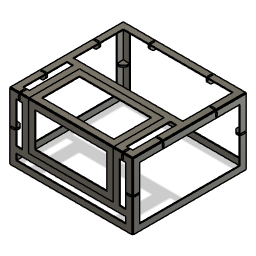
Frameoko_V1.0.0 (Autodesk Fusion 360 design; units mm, degrees)
Autodesk Fusion 360 part; units mm, degrees
(part 1 of 3)
sketch "machine_footprint" plane through (0, 0, 0) normal (0, 1, 0) x (1, 0, 0)
  line L0 (495.3, 457.2) -> (-495.3, 457.2)
  line L1 (-495.3, 457.2) -> (-495.3, -457.2)
  line L2 (-495.3, -457.2) -> (495.3, -457.2)
  line L3 (495.3, -457.2) -> (495.3, 457.2)
  line L4 (495.3, 457.2) -> (-495.3, -457.2) construction
  line L5 (-495.3, 457.2) -> (495.3, -457.2) construction
  dimension "d4" = 990.6
  dimension "d5" = 914.4
  constraint horizontal L0
  constraint perpendicular L0 L1
  constraint parallel L0 L2
  constraint parallel L1 L3
  constraint coincident L4 origin
  constraint coincident L5 origin
  measures "d4" distance of L1.end L2.end
  measures "d5" distance of L0.end L1.end
extrude "Extrude1" add sketch "machine_footprint" along normal mid plane 533.4 makes body 1
sketch "back-face" plane through (0, 0, 0) normal (0, 0, 1) x (1, 0, 0)
  line L0 (495.3, 266.7) -> (-495.3, 266.7)
  line L1 (-495.3, 266.7) -> (-495.3, -266.7)
  line L2 (-495.3, -266.7) -> (495.3, -266.7)
  line L3 (495.3, -266.7) -> (495.3, 266.7)
  line L4 (495.3, 266.7) -> (-495.3, -266.7) construction
  line L5 (-495.3, 266.7) -> (495.3, -266.7) construction
  line L6 (444.5, 215.9) -> (-444.5, 215.9)
  line L7 (-444.5, 215.9) -> (-444.5, -215.9)
  line L8 (-444.5, -215.9) -> (444.5, -215.9)
  line L9 (444.5, -215.9) -> (444.5, 215.9)
  line L10 (444.5, 215.9) -> (-444.5, -215.9) construction
  line L11 (-444.5, 215.9) -> (444.5, -215.9) construction
  line L12 (-495.3, 266.7) -> (-444.5, 266.7)
  line L13 (-444.5, 266.7) -> (-444.5, 215.9)
  line L14 (-444.5, 215.9) -> (-495.3, 215.9)
  line L15 (-495.3, 215.9) -> (-495.3, 266.7)
  line L16 (495.3, 266.7) -> (444.5, 266.7)
  line L17 (444.5, 266.7) -> (444.5, 215.9)
  line L18 (444.5, 215.9) -> (495.3, 215.9)
  line L19 (495.3, 215.9) -> (495.3, 266.7)
  line L20 (495.3, -266.7) -> (444.5, -266.7)
  line L21 (444.5, -266.7) -> (444.5, -215.9)
  line L22 (444.5, -215.9) -> (495.3, -215.9)
  line L23 (495.3, -215.9) -> (495.3, -266.7)
  line L24 (-495.3, -266.7) -> (-444.5, -266.7)
  line L25 (-444.5, -266.7) -> (-444.5, -215.9)
  line L26 (-444.5, -215.9) -> (-495.3, -215.9)
  line L27 (-495.3, -215.9) -> (-495.3, -266.7)
  line L28 (-444.5, 266.7) -> (-444.5, 215.9)
  line L29 (-444.5, 215.9) -> (-393.7, 215.9)
  line L30 (-393.7, 215.9) -> (-393.7, 266.7)
  line L31 (-393.7, 266.7) -> (-444.5, 266.7)
  line L32 (444.5, 266.7) -> (444.5, 215.9)
  line L33 (444.5, 215.9) -> (393.7, 215.9)
  line L34 (393.7, 215.9) -> (393.7, 266.7)
  line L35 (393.7, 266.7) -> (444.5, 266.7)
  line L36 (-444.5, 215.9) -> (-495.3, 215.9)
  line L37 (-495.3, 215.9) -> (-495.3, 165.1)
  line L38 (-495.3, 165.1) -> (-444.5, 165.1)
  line L39 (-444.5, 165.1) -> (-444.5, 215.9)
  line L40 (495.3, 215.9) -> (444.5, 215.9)
  line L41 (444.5, 215.9) -> (444.5, 165.1)
  line L42 (444.5, 165.1) -> (495.3, 165.1)
  line L43 (495.3, 165.1) -> (495.3, 215.9)
  line L44 (495.3, -215.9) -> (444.5, -215.9)
  line L45 (444.5, -215.9) -> (444.5, -165.1)
  line L46 (444.5, -165.1) -> (495.3, -165.1)
  line L47 (495.3, -165.1) -> (495.3, -215.9)
  line L48 (444.5, -215.9) -> (444.5, -266.7)
  line L49 (444.5, -266.7) -> (393.7, -266.7)
  line L50 (393.7, -266.7) -> (393.7, -215.9)
  line L51 (393.7, -215.9) -> (444.5, -215.9)
  line L52 (-444.5, -215.9) -> (-444.5, -266.7)
  line L53 (-444.5, -266.7) -> (-393.7, -266.7)
  line L54 (-393.7, -266.7) -> (-393.7, -215.9)
  line L55 (-393.7, -215.9) -> (-444.5, -215.9)
  line L56 (-444.5, -215.9) -> (-495.3, -215.9)
  line L57 (-495.3, -215.9) -> (-495.3, -165.1)
  line L58 (-495.3, -165.1) -> (-444.5, -165.1)
  line L59 (-444.5, -165.1) -> (-444.5, -215.9)
  line L60 (444.5, 266.7) -> (393.7, 215.9)
  line L61 (495.3, 215.9) -> (444.5, 165.1)
  line L62 (495.3, -215.9) -> (444.5, -165.1)
  line L63 (393.7, -215.9) -> (444.5, -266.7)
  line L64 (-444.5, -266.7) -> (-393.7, -215.9)
  line L65 (-495.3, -215.9) -> (-444.5, -165.1)
  line L66 (-444.5, 266.7) -> (-393.7, 215.9)
  line L67 (-495.3, 215.9) -> (-444.5, 165.1)
  circle A0 centre (-419.1, 241.3) radius 15.875
  circle A1 centre (419.1, 241.3) radius 15.875
  circle A2 centre (469.9, 190.5) radius 15.875
  circle A3 centre (469.9, -190.5) radius 15.875
  circle A4 centre (419.1, -241.3) radius 15.875
  circle A5 centre (-419.1, -241.3) radius 15.875
  circle A6 centre (-469.9, -190.5) radius 15.875
  circle A7 centre (-469.9, 190.5) radius 15.875
  line L68 (-165.1, 266.7) -> (-165.1, 215.9)
  circle A8 centre (-139.7, 241.3) radius 15.875
  line L69 (-114.3, 215.9) -> (-114.3, 266.7)
  line L70 (114.3, 266.7) -> (114.3, 215.9)
  circle A9 centre (139.7, 241.3) radius 15.875
  line L71 (165.1, 215.9) -> (165.1, 266.7)
  circle A10 centre (469.9, -190.5) radius 15.875
  line L72 (495.3, -165.1) -> (444.5, -165.1)
  line L73 (444.5, -215.9) -> (495.3, -215.9)
  line L74 (393.7, 266.7) -> (393.7, 215.9)
  circle A11 centre (419.1, 241.3) radius 15.875
  line L75 (444.5, 215.9) -> (444.5, 266.7)
  circle A12 centre (-469.9, -190.5) radius 15.875
  line L76 (-495.3, -215.9) -> (-444.5, -215.9)
  line L77 (-444.5, -165.1) -> (-495.3, -165.1)
  circle A13 centre (-139.7, -241.3) radius 15.875
  line L78 (-114.3, -266.7) -> (-114.3, -215.9)
  line L79 (-165.1, -266.7) -> (-165.1, -215.9)
  circle A14 centre (139.7, -241.3) radius 15.875
  line L80 (165.1, -266.7) -> (165.1, -215.9)
  line L81 (114.3, -266.7) -> (114.3, -215.9)
  circle A15 centre (419.1, -241.3) radius 15.875
  line L82 (444.5, -266.7) -> (444.5, -215.9)
  line L83 (393.7, -266.7) -> (393.7, -215.9)
  dimension "d49" = 990.6
  dimension "d50" = 533.4
  dimension "d51" = 889
  dimension "d52" = 431.8
  dimension "d259" = 50.8
  dimension "d260" = 50.8
  dimension "d261" = 50.8
  dimension "d262" = 50.8
  dimension "d263" = 50.8
  dimension "d264" = 50.8
  dimension "d265" = 50.8
  dimension "d266" = 50.8
  dimension "d267" = 50.8
  dimension "d268" = 50.8
  dimension "d269" = 50.8
  dimension "d270" = 50.8
  dimension "d271" = 50.8
  dimension "d272" = 50.8
  dimension "d273" = 50.8
  dimension "d274" = 50.8
  dimension "d275" = 31.75
  dimension "d276" = 31.75
  dimension "d277" = 31.75
  dimension "d278" = 31.75
  dimension "d279" = 31.75
  dimension "d280" = 31.75
  dimension "d281" = 31.75
  dimension "d282" = 31.75
  dimension "d285" = 838.2
  dimension "d286" = 0
  dimension "d297" = 0
  dimension "d298" = -381
  constraint horizontal L0
  constraint perpendicular L0 L1
  constraint parallel L0 L2
  constraint parallel L1 L3
  constraint coincident L4 origin
  constraint coincident L5 origin
  constraint horizontal L6
  constraint perpendicular L6 L7
  constraint parallel L6 L8
  constraint parallel L7 L9
  constraint coincident L10 origin
  constraint coincident L11 origin
  constraint horizontal L12
  constraint vertical L13
  constraint horizontal L14
  constraint vertical L15
  constraint horizontal L16
  constraint vertical L17
  constraint horizontal L18
  constraint vertical L19
  constraint horizontal L20
  constraint vertical L21
  constraint horizontal L22
  constraint vertical L23
  constraint horizontal L24
  constraint vertical L25
  constraint horizontal L26
  constraint vertical L27
  constraint perpendicular L28 L29
  constraint parallel L28 L30
  constraint parallel L29 L31
  constraint perpendicular L32 L33
  constraint parallel L32 L34
  constraint parallel L33 L35
  constraint perpendicular L36 L37
  constraint parallel L36 L38
  constraint parallel L37 L39
  constraint perpendicular L40 L41
  constraint parallel L40 L42
  constraint parallel L41 L43
  constraint perpendicular L44 L45
  constraint parallel L44 L46
  constraint parallel L45 L47
  constraint perpendicular L48 L49
  constraint parallel L48 L50
  constraint parallel L49 L51
  constraint perpendicular L52 L53
  constraint parallel L52 L54
  constraint parallel L53 L55
  constraint perpendicular L56 L57
  constraint parallel L56 L58
  constraint parallel L57 L59
  constraint midpoint L66 A0.centre
  constraint midpoint L60 A1.centre
  constraint midpoint L61 A2.centre
  constraint midpoint L62 A3.centre
  constraint midpoint L63 A4.centre
  constraint midpoint L64 A5.centre
  constraint midpoint L65 A6.centre
  constraint midpoint L67 A7.centre
  measures "d49" distance of L1.end L2.end
  measures "d50" distance of L0.end L1.end
  measures "d51" distance of L7.end L8.end
  measures "d52" distance of L6.end L7.end
  measures "d259" distance of L0.end L12.end
  measures "d260" distance of L0.end L14.end
  measures "d261" distance of L0.start L16.end
  measures "d262" distance of L0.start L18.end
  measures "d263" distance of L2.end L20.end
  measures "d264" distance of L2.end L22.end
  measures "d265" distance of L1.end L24.end
  measures "d266" distance of L1.end L26.end
  measures "d267" distance of L12.end L30.end
  measures "d268" distance of L16.end L34.end
  measures "d269" distance of L6.end L38.end
  measures "d270" distance of L18.end L42.end
  measures "d271" distance of L22.end L46.end
  measures "d272" distance of L8.end L50.end
  measures "d273" distance of L7.end L54.end
  measures "d274" distance of L7.end L58.end
  measures "d275" diameter of A0
  measures "d276" diameter of A1
  measures "d277" diameter of A2
  measures "d278" diameter of A3
  measures "d279" diameter of A4
  measures "d280" diameter of A5
  measures "d281" diameter of A6
  measures "d282" diameter of A7
extrude "Extrude9" add sketch "back-face" along normal blind -457.2 and the other way blind 463.55 separate body contours L0 L3 L16 L17 L18 L19 L32 L40 L75 | L0 L34 L35 L60 A1 L74 A11 | L6 L17 L32 L33 L60 A1 A11 L75 | L9 L18 L40 L41 L61 A2 | L3 L42 L43 L61 A2 | L0 L6 L34 L71 L74 | L60 A1 A11 | L60 A1 A11 | L3 L9 L42 L46 L72 | L61 A2 | L61 A2 | L0 L6 L70 L71 | L3 L46 L47 L62 A3 A10 L72 | L0 L6 L69 L70 | L9 L22 L44 L45 L62 A3 A10 L73 | L2 L3 L20 L21 L22 L23 L44 L48 L73 L82 | L0 L6 L68 L69 | L8 L21 L48 L51 L63 A4 A15 L82 | L62 A3 A10 | L62 A3 A10 | L0 L6 L30 L68 | L2 L8 L50 L80 L83 | L2 L49 L50 L63 A4 A15 L83 | L0 L30 L31 L66 A0 | L2 L8 L80 L81 | L63 A4 A15 | L63 A4 A15 | L0 L1 L12 L13 L14 L15 L28 L36 | L6 L13 L28 L29 L66 A0 | L2 L8 L78 L81 | L7 L14 L36 L39 L67 A7 | L66 A0 | L66 A0 | L2 L8 L78 L79 | L1 L37 L38 L67 A7 | L1 L7 L38 L58 L77 | L2 L8 L54 L79 | L67 A7 | L67 A7 | L1 L57 L58 L65 A6 A12 L77 | L7 L26 L56 L59 L65 A6 A12 L76 | L8 L25 L52 L55 L64 A5 | L2 L53 L54 L64 A5 | L1 L2 L24 L25 L26 L27 L52 L56 L76 | L65 A6 A12 | L65 A6 A12 | L64 A5 | L64 A5 | A8 | A9 | A13 | A14 makes body 2
sketch "LR-faces" plane through (0, 0, 0) normal (1, 0, 0) x (0, 0, -1)
  line L0 (457.2, 266.7) -> (-457.2, 266.7)
  line L1 (-457.2, 266.7) -> (-457.2, -266.7)
  line L2 (-457.2, -266.7) -> (457.2, -266.7)
  line L3 (457.2, -266.7) -> (457.2, 266.7)
  line L4 (457.2, 266.7) -> (-457.2, -266.7) construction
  line L5 (-457.2, 266.7) -> (457.2, -266.7) construction
  line L6 (406.4, 215.9) -> (-406.4, 215.9)
  line L7 (-406.4, 215.9) -> (-406.4, -215.9)
  line L8 (-406.4, -215.9) -> (406.4, -215.9)
  line L9 (406.4, -215.9) -> (406.4, 215.9)
  line L10 (406.4, 215.9) -> (-406.4, -215.9) construction
  line L11 (-406.4, 215.9) -> (406.4, -215.9) construction
  line L12 (-457.2, 266.7) -> (-406.4, 266.7)
  line L13 (-406.4, 266.7) -> (-406.4, 215.9)
  line L14 (-406.4, 215.9) -> (-457.2, 215.9)
  line L15 (-457.2, 215.9) -> (-457.2, 266.7)
  line L16 (457.2, 266.7) -> (406.4, 266.7)
  line L17 (406.4, 266.7) -> (406.4, 215.9)
  line L18 (406.4, 215.9) -> (457.2, 215.9)
  line L19 (457.2, 215.9) -> (457.2, 266.7)
  line L20 (457.2, -266.7) -> (406.4, -266.7)
  line L21 (406.4, -266.7) -> (406.4, -215.9)
  line L22 (406.4, -215.9) -> (457.2, -215.9)
  line L23 (457.2, -215.9) -> (457.2, -266.7)
  line L24 (-457.2, -266.7) -> (-406.4, -266.7)
  line L25 (-406.4, -266.7) -> (-406.4, -215.9)
  line L26 (-406.4, -215.9) -> (-457.2, -215.9)
  line L27 (-457.2, -215.9) -> (-457.2, -266.7)
  line L28 (-406.4, 266.7) -> (-406.4, 215.9)
  line L29 (-406.4, 215.9) -> (-355.6, 215.9)
  line L30 (-355.6, 215.9) -> (-355.6, 266.7)
  line L31 (-355.6, 266.7) -> (-406.4, 266.7)
  line L32 (406.4, 266.7) -> (406.4, 215.9)
  line L33 (406.4, 215.9) -> (355.6, 215.9)
  line L34 (355.6, 215.9) -> (355.6, 266.7)
  line L35 (355.6, 266.7) -> (406.4, 266.7)
  line L36 (-406.4, 266.7) -> (-355.6, 215.9)
  circle A0 centre (-381, 241.3) radius 15.875
  line L37 (355.6, 266.7) -> (406.4, 215.9)
  circle A1 centre (381, 241.3) radius 15.875
  circle A2 centre (-127, 241.3) radius 15.875
  line L38 (-101.6, 215.9) -> (-101.6, 266.7)
  line L39 (-152.4, 266.7) -> (-152.4, 215.9)
  line L40 (-406.4, -215.9) -> (-406.4, -266.7)
  line L41 (-406.4, -266.7) -> (-355.6, -266.7)
  line L42 (-355.6, -266.7) -> (-355.6, -215.9)
  line L43 (-355.6, -215.9) -> (-406.4, -215.9)
  line L44 (406.4, -215.9) -> (406.4, -266.7)
  line L45 (406.4, -266.7) -> (355.6, -266.7)
  line L46 (355.6, -266.7) -> (355.6, -215.9)
  line L47 (355.6, -215.9) -> (406.4, -215.9)
  line L48 (355.6, -215.9) -> (406.4, -266.7)
  line L49 (-406.4, -215.9) -> (-355.6, -266.7)
  line L50 (-406.4, 215.9) -> (-457.2, 215.9)
  line L51 (-457.2, 215.9) -> (-457.2, 165.1)
  line L52 (-457.2, 165.1) -> (-406.4, 165.1)
  line L53 (-406.4, 165.1) -> (-406.4, 215.9)
  line L54 (-406.4, -215.9) -> (-457.2, -215.9)
  line L55 (-457.2, -215.9) -> (-457.2, -165.1)
  line L56 (-457.2, -165.1) -> (-406.4, -165.1)
  line L57 (-406.4, -165.1) -> (-406.4, -215.9)
  line L58 (-457.2, 215.9) -> (-406.4, 165.1)
  circle A3 centre (-431.8, 190.5) radius 15.875
  circle A4 centre (-381, -241.3) radius 15.875
  circle A5 centre (381, -241.3) radius 15.875
  line L59 (406.4, 215.9) -> (457.2, 215.9)
  line L60 (457.2, 215.9) -> (457.2, 165.1)
  line L61 (457.2, 165.1) -> (406.4, 165.1)
  line L62 (406.4, 165.1) -> (406.4, 215.9)
  line L63 (457.2, -215.9) -> (406.4, -215.9)
  line L64 (406.4, -215.9) -> (406.4, -165.1)
  line L65 (406.4, -165.1) -> (457.2, -165.1)
  line L66 (457.2, -165.1) -> (457.2, -215.9)
  line L67 (406.4, -165.1) -> (457.2, -215.9)
  circle A6 centre (431.8, -190.5) radius 15.875
  line L68 (406.4, 165.1) -> (457.2, 215.9)
  circle A7 centre (431.8, 190.5) radius 15.875
  line L69 (-406.4, -165.1) -> (-457.2, -215.9)
  circle A8 centre (-431.8, -190.5) radius 15.875
  line L70 (-457.2, -215.9) -> (-406.4, -215.9)
  line L71 (-406.4, -165.1) -> (-457.2, -165.1)
  circle A9 centre (-431.8, -190.5) radius 15.875
  circle A10 centre (-127, -241.3) radius 15.875
  line L72 (-152.4, -215.9) -> (-152.4, -266.7)
  line L73 (-101.6, -266.7) -> (-101.6, -215.9)
  circle A11 centre (431.8, -190.5) radius 15.875
  line L74 (406.4, -165.1) -> (457.2, -165.1)
  line L75 (457.2, -215.9) -> (406.4, -215.9)
  circle A12 centre (127, 241.3) radius 15.875
  line L76 (152.4, 215.9) -> (152.4, 266.7)
  line L77 (101.6, 266.7) -> (101.6, 215.9)
  circle A13 centre (127, -241.3) radius 15.875
  line L78 (101.6, -215.9) -> (101.6, -266.7)
  line L79 (152.4, -266.7) -> (152.4, -215.9)
  circle A14 centre (381, 241.3) radius 15.875
  line L80 (406.4, 215.9) -> (406.4, 266.7)
  line L81 (355.6, 266.7) -> (355.6, 215.9)
  circle A15 centre (381, -241.3) radius 15.875
  line L82 (355.6, -215.9) -> (355.6, -266.7)
  line L83 (406.4, -266.7) -> (406.4, -215.9)
  point P0 (0, 292.1)
  point P1 (431.8, 0)
  point P2 (-431.8, 0)
  dimension "d81" = 914.4
  dimension "d82" = 533.4
  dimension "d83" = 812.8
  dimension "d84" = 431.8
  dimension "d202" = 50.8
  dimension "d203" = 50.8
  dimension "d204" = 50.8
  dimension "d205" = 50.8
  dimension "d206" = 50.8
  dimension "d207" = 50.8
  dimension "d208" = 50.8
  dimension "d209" = 50.8
  dimension "d210" = 50.8
  dimension "d211" = 50.8
  dimension "d212" = 31.75
  dimension "d213" = 31.75
  dimension "d216" = 762
  dimension "d217" = 0
  dimension "d218" = 50.8
  dimension "d219" = 50.8
  dimension "d220" = 50.8
  dimension "d221" = 50.8
  dimension "d222" = 31.75
  dimension "d224" = 31.75
  dimension "d225" = 31.75
  dimension "d226" = 50.8
  dimension "d227" = 50.8
  dimension "d229" = 31.75
  dimension "d230" = 31.75
  dimension "d231" = 31.75
  dimension "d239" = 0
  dimension "d240" = -381
  constraint horizontal L0
  constraint perpendicular L0 L1
  constraint parallel L0 L2
  constraint parallel L1 L3
  constraint coincident L4 origin
  constraint coincident L5 origin
  constraint horizontal L6
  constraint perpendicular L6 L7
  constraint parallel L6 L8
  constraint parallel L7 L9
  constraint coincident L10 origin
  constraint coincident L11 origin
  constraint horizontal L12
  constraint vertical L13
  constraint horizontal L14
  constraint vertical L15
  constraint horizontal L16
  constraint vertical L17
  constraint horizontal L18
  constraint vertical L19
  constraint horizontal L20
  constraint vertical L21
  constraint horizontal L22
  constraint vertical L23
  constraint horizontal L24
  constraint vertical L25
  constraint horizontal L26
  constraint vertical L27
  constraint perpendicular L28 L29
  constraint parallel L28 L30
  constraint parallel L29 L31
  constraint perpendicular L32 L33
  constraint parallel L32 L34
  constraint parallel L33 L35
  constraint midpoint L36 A0.centre
  constraint midpoint L37 A1.centre
  constraint perpendicular L40 L41
  constraint parallel L40 L42
  constraint parallel L41 L43
  constraint perpendicular L44 L45
  constraint parallel L44 L46
  constraint parallel L45 L47
  constraint perpendicular L50 L51
  constraint parallel L50 L52
  constraint parallel L51 L53
  constraint perpendicular L54 L55
  constraint parallel L54 L56
  constraint parallel L55 L57
  constraint midpoint L58 A3.centre
  constraint midpoint L49 A4.centre
  constraint midpoint L48 A5.centre
  constraint perpendicular L59 L60
  constraint parallel L59 L61
  constraint parallel L60 L62
  constraint perpendicular L63 L64
  constraint parallel L63 L65
  constraint parallel L64 L66
  constraint midpoint L67 A6.centre
  constraint midpoint L68 A7.centre
  constraint midpoint L69 A8.centre
  measures "d81" distance of L1.end L2.end
  measures "d82" distance of L0.end L1.end
  measures "d83" distance of L7.end L8.end
  measures "d84" distance of L6.end L7.end
  measures "d202" distance of L0.end L12.end
  measures "d203" distance of L0.end L14.end
  measures "d204" distance of L0.start L16.end
  measures "d205" distance of L0.start L18.end
  measures "d206" distance of L2.end L20.end
  measures "d207" distance of L2.end L22.end
  measures "d208" distance of L1.end L24.end
  measures "d209" distance of L1.end L26.end
  measures "d210" distance of L12.end L30.end
  measures "d211" distance of L16.end L34.end
  measures "d212" diameter of A0
  measures "d213" diameter of A1
  measures "d218" distance of L7.end L42.end
  measures "d219" distance of L8.end L46.end
  measures "d220" distance of L6.end L52.end
  measures "d221" distance of L7.end L56.end
  measures "d222" diameter of A3
  measures "d224" diameter of A4
  measures "d225" diameter of A5
  measures "d226" distance of L6.start L61.end
  measures "d227" distance of L22.end L65.end
  measures "d229" diameter of A6
  measures "d230" diameter of A7
  measures "d231" diameter of A8
extrude "Extrude13" add sketch "LR-faces" along normal blind 501.65 and the other way blind -495.3 separate body contours L0 L3 L16 L17 L18 L19 L32 L59 L80 | L0 L17 L32 L35 L37 A1 A14 L80 | L9 L18 L59 L62 L68 A7 | L3 L60 L61 L68 A7 | L0 L6 L34 L76 L81 | L6 L33 L34 L37 A1 A14 L81 | L3 L9 L61 L65 L74 | L68 A7 | L68 A7 | L0 L6 L76 L77 | L37 A1 A14 | L37 A1 A14 | L3 L65 L66 L67 A6 A11 L74 | L0 L6 L38 L77 | L9 L22 L63 L64 L67 A6 A11 L75 | L2 L3 L20 L21 L22 L23 L44 L63 L75 L83 | L0 L6 L38 L39 | L8 L21 L44 L47 L48 A5 A15 L83 | L67 A6 A11 | L67 A6 A11 | L0 L6 L30 L39 | L2 L8 L46 L79 L82 | L2 L45 L46 L48 A5 A15 L82 | L0 L30 L31 L36 A0 | L2 L8 L78 L79 | L48 A5 A15 | L48 A5 A15 | L0 L1 L12 L13 L14 L15 L28 L50 | L6 L13 L28 L29 L36 A0 | L2 L8 L73 L78 | L7 L14 L50 L53 L58 A3 | L36 A0 | L36 A0 | L2 L8 L72 L73 | L1 L51 L52 L58 A3 | L1 L7 L52 L56 L71 | L2 L8 L42 L72 | L58 A3 | L58 A3 | L1 L55 L56 L69 A8 L71 A9 | L7 L26 L54 L57 L69 A8 L70 A9 | L8 L42 L43 L49 A4 | L2 L25 L40 L41 L49 A4 | L1 L2 L24 L25 L26 L27 L40 L54 L70 | L69 A8 A9 | L69 A8 A9 | L49 A4 | L49 A4 | A2 | A10 | A12 | A13 makes body 3
extrude "Extrude14" add sketch "LR-faces" along normal blind -501.65 and the other way blind 495.3 separate body contours L0 L3 L16 L17 L18 L19 L32 L59 L80 | L0 L17 L32 L35 L37 A1 A14 L80 | L9 L18 L59 L62 L68 A7 | L3 L60 L61 L68 A7 | L0 L6 L34 L76 L81 | L6 L33 L34 L37 A1 A14 L81 | L3 L9 L61 L65 L74 | L68 A7 | L68 A7 | L0 L6 L76 L77 | L37 A1 A14 | L37 A1 A14 | L3 L65 L66 L67 A6 A11 L74 | L0 L6 L38 L77 | L9 L22 L63 L64 L67 A6 A11 L75 | L2 L3 L20 L21 L22 L23 L44 L63 L75 L83 | L0 L6 L38 L39 | L8 L21 L44 L47 L48 A5 A15 L83 | L67 A6 A11 | L67 A6 A11 | L0 L6 L30 L39 | L2 L8 L46 L79 L82 | L2 L45 L46 L48 A5 A15 L82 | L0 L30 L31 L36 A0 | L2 L8 L78 L79 | L48 A5 A15 | L48 A5 A15 | L0 L1 L12 L13 L14 L15 L28 L50 | L6 L13 L28 L29 L36 A0 | L2 L8 L73 L78 | L7 L14 L50 L53 L58 A3 | L36 A0 | L36 A0 | L2 L8 L72 L73 | L1 L51 L52 L58 A3 | L1 L7 L52 L56 L71 | L2 L8 L42 L72 | L58 A3 | L58 A3 | L1 L55 L56 L69 A8 L71 A9 | L7 L26 L54 L57 L69 A8 L70 A9 | L8 L42 L43 L49 A4 | L2 L25 L40 L41 L49 A4 | L1 L2 L24 L25 L26 L27 L40 L54 L70 | L69 A8 A9 | L69 A8 A9 | L49 A4 | L49 A4 | A2 | A10 | A12 | A13 makes body 4
sketch "top-face" plane through (0, 0, 0) normal (0, 1, 0) x (1, 0, 0)
  line L0 (495.3, -457.2) -> (-495.3, -457.2)
  line L1 (-495.3, -457.2) -> (-495.3, 457.2)
  line L2 (-495.3, 457.2) -> (495.3, 457.2)
  line L3 (495.3, 457.2) -> (495.3, -457.2)
  line L4 (495.3, -457.2) -> (-495.3, 457.2) construction
  line L5 (-495.3, -457.2) -> (495.3, 457.2) construction
  line L6 (495.3, -457.2) -> (342.9, -457.2)
  line L7 (342.9, -457.2) -> (342.9, -50.8)
  line L8 (342.9, -50.8) -> (495.3, -50.8)
  line L9 (495.3, -50.8) -> (495.3, -457.2)
  line L10 (-495.3, -457.2) -> (-342.9, -457.2)
  line L11 (-342.9, -457.2) -> (-342.9, -50.8)
  line L12 (-342.9, -50.8) -> (-495.3, -50.8)
  line L13 (-495.3, -50.8) -> (-495.3, -457.2)
  line L14 (-495.3, -50.8) -> (495.3, -50.8)
  line L15 (495.3, -50.8) -> (495.3, 0)
  line L16 (495.3, 0) -> (-495.3, 0)
  line L17 (-495.3, 0) -> (-495.3, -50.8)
  line L18 (-495.3, 457.2) -> (495.3, 457.2)
  line L19 (495.3, 457.2) -> (495.3, 406.4)
  line L20 (495.3, 406.4) -> (-495.3, 406.4)
  line L21 (-495.3, 406.4) -> (-495.3, 457.2)
  line L22 (495.3, -457.2) -> (342.9, -457.2)
  line L23 (342.9, -457.2) -> (342.9, -406.4)
  line L24 (342.9, -406.4) -> (495.3, -406.4)
  line L25 (495.3, -406.4) -> (495.3, -457.2)
  line L26 (-495.3, -457.2) -> (-342.9, -457.2)
  line L27 (-342.9, -457.2) -> (-342.9, -406.4)
  line L28 (-342.9, -406.4) -> (-495.3, -406.4)
  line L29 (-495.3, -406.4) -> (-495.3, -457.2)
  line L30 (495.3, -457.2) -> (495.3, 457.2)
  line L31 (495.3, 457.2) -> (444.5, 457.2)
  line L32 (444.5, 457.2) -> (444.5, -457.2)
  line L33 (444.5, -457.2) -> (495.3, -457.2)
  line L34 (-495.3, 457.2) -> (-495.3, -457.2)
  line L35 (-495.3, -457.2) -> (-444.5, -457.2)
  line L36 (-444.5, -457.2) -> (-444.5, 457.2)
  line L37 (-444.5, 457.2) -> (-495.3, 457.2)
  line L38 (-342.9, -457.2) -> (-342.9, -50.8)
  line L39 (-342.9, -50.8) -> (-393.7, -50.8)
  line L40 (-393.7, -50.8) -> (-393.7, -457.2)
  line L41 (-393.7, -457.2) -> (-342.9, -457.2)
  line L42 (342.9, -457.2) -> (342.9, -50.8)
  line L43 (342.9, -50.8) -> (393.7, -50.8)
  line L44 (393.7, -50.8) -> (393.7, -457.2)
  line L45 (393.7, -457.2) -> (342.9, -457.2)
  line L46 (-342.9, -457.2) -> (342.9, -457.2)
  line L47 (342.9, -457.2) -> (342.9, -406.4)
  line L48 (342.9, -406.4) -> (-342.9, -406.4)
  line L49 (-342.9, -406.4) -> (-342.9, -457.2)
  line L50 (-342.9, -50.8) -> (342.9, -50.8)
  line L51 (342.9, -50.8) -> (342.9, -101.6)
  line L52 (342.9, -101.6) -> (-342.9, -101.6)
  line L53 (-342.9, -101.6) -> (-342.9, -50.8)
  line L54 (-342.9, -50.8) -> (-342.9, -457.2)
  line L55 (-342.9, -457.2) -> (-292.1, -457.2)
  line L56 (-292.1, -457.2) -> (-292.1, -50.8)
  line L57 (-292.1, -50.8) -> (-342.9, -50.8)
  line L58 (342.9, -50.8) -> (342.9, -457.2)
  line L59 (342.9, -457.2) -> (292.1, -457.2)
  line L60 (292.1, -457.2) -> (292.1, -50.8)
  line L61 (292.1, -50.8) -> (342.9, -50.8)
  line L62 (-342.9, -406.4) -> (-292.1, -406.4)
  line L63 (-292.1, -406.4) -> (-292.1, -355.6)
  line L64 (-292.1, -355.6) -> (-342.9, -355.6)
  line L65 (-342.9, -355.6) -> (-342.9, -406.4)
  line L66 (342.9, -406.4) -> (292.1, -406.4)
  line L67 (292.1, -406.4) -> (292.1, -355.6)
  line L68 (292.1, -355.6) -> (342.9, -355.6)
  line L69 (342.9, -355.6) -> (342.9, -406.4)
  line L70 (-342.9, -355.6) -> (-292.1, -406.4)
  circle A0 centre (-317.5, -381) radius 15.875
  line L71 (342.9, -355.6) -> (292.1, -406.4)
  circle A1 centre (317.5, -381) radius 15.875
  circle A2 centre (-317.5, -127) radius 15.875
  line L72 (-292.1, -101.6) -> (-342.9, -101.6)
  circle A3 centre (317.5, -127) radius 15.875
  line L73 (292.1, -101.6) -> (342.9, -101.6)
  line L74 (342.9, -152.4) -> (292.1, -152.4)
  line L75 (-342.9, -152.4) -> (-292.1, -152.4)
  line L76 (-292.1, -50.8) -> (-292.1, -101.6)
  line L77 (-292.1, -101.6) -> (-241.3, -101.6)
  line L78 (-241.3, -101.6) -> (-241.3, -50.8)
  line L79 (-241.3, -50.8) -> (-292.1, -50.8)
  line L80 (-292.1, -406.4) -> (-292.1, -457.2)
  line L81 (-292.1, -457.2) -> (-241.3, -457.2)
  line L82 (-241.3, -457.2) -> (-241.3, -406.4)
  line L83 (-241.3, -406.4) -> (-292.1, -406.4)
  line L84 (-292.1, -457.2) -> (-241.3, -406.4)
  line L85 (-292.1, -50.8) -> (-241.3, -101.6)
  circle A4 centre (-266.7, -76.2) radius 15.875
  circle A5 centre (-266.7, -431.8) radius 15.875
  circle A6 centre (-88.9, -431.8) radius 15.875
  circle A7 centre (-88.9, -76.2) radius 15.875
  line L86 (-63.5, -101.6) -> (-63.5, -50.8)
  line L87 (-63.5, -457.2) -> (-63.5, -406.4)
  line L88 (-114.3, -406.4) -> (-114.3, -457.2)
  line L89 (-114.3, -50.8) -> (-114.3, -101.6)
  circle A8 centre (88.9, -431.8) radius 15.875
  circle A9 centre (88.9, -76.2) radius 15.875
  line L90 (114.3, -101.6) -> (114.3, -50.8)
  line L91 (114.3, -457.2) -> (114.3, -406.4)
  line L92 (63.5, -406.4) -> (63.5, -457.2)
  line L93 (63.5, -50.8) -> (63.5, -101.6)
  circle A10 centre (266.7, -431.8) radius 15.875
  circle A11 centre (266.7, -76.2) radius 15.875
  line L94 (292.1, -101.6) -> (292.1, -50.8)
  line L95 (292.1, -457.2) -> (292.1, -406.4)
  line L96 (241.3, -406.4) -> (241.3, -457.2)
  line L97 (241.3, -50.8) -> (241.3, -101.6)
  line L98 (-444.5, 457.2) -> (-444.5, 406.4)
  line L99 (-444.5, 406.4) -> (-393.7, 406.4)
  line L100 (-393.7, 406.4) -> (-393.7, 457.2)
  line L101 (-393.7, 457.2) -> (-444.5, 457.2)
  line L102 (-444.5, 457.2) -> (-393.7, 406.4)
  circle A12 centre (-419.1, 431.8) radius 15.875
  circle A13 centre (-139.7, 431.8) radius 15.875
  line L103 (-114.3, 406.4) -> (-114.3, 457.2)
  line L104 (-165.1, 457.2) -> (-165.1, 406.4)
  circle A14 centre (139.7, 431.8) radius 15.875
  line L105 (165.1, 406.4) -> (165.1, 457.2)
  line L106 (114.3, 457.2) -> (114.3, 406.4)
  circle A15 centre (419.1, 431.8) radius 15.875
  line L107 (444.5, 406.4) -> (444.5, 457.2)
  line L108 (393.7, 457.2) -> (393.7, 406.4)
  line L109 (444.5, 406.4) -> (495.3, 406.4)
  line L110 (495.3, 406.4) -> (495.3, 355.6)
  line L111 (495.3, 355.6) -> (444.5, 355.6)
  line L112 (444.5, 355.6) -> (444.5, 406.4)
  line L113 (444.5, 406.4) -> (495.3, 355.6)
  circle A16 centre (469.9, 381) radius 15.875
  line L114 (-495.3, 406.4) -> (-444.5, 406.4)
  line L115 (-444.5, 406.4) -> (-444.5, 355.6)
  line L116 (-444.5, 355.6) -> (-495.3, 355.6)
  line L117 (-495.3, 355.6) -> (-495.3, 406.4)
  line L118 (-444.5, 406.4) -> (-495.3, 355.6)
  circle A17 centre (-469.9, 381) radius 15.875
  circle A18 centre (469.9, 25.4) radius 15.875
  line L119 (495.3, 0) -> (444.5, 0)
  circle A19 centre (-469.9, 25.4) radius 15.875
  line L120 (-444.5, 0) -> (-495.3, 0)
  line L121 (-444.5, 50.8) -> (-444.5, 0)
  line L122 (-495.3, 0) -> (-495.3, 50.8)
  line L123 (444.5, 0) -> (444.5, 50.8)
  line L124 (495.3, 50.8) -> (495.3, 0)
  line L125 (444.5, 50.8) -> (495.3, 50.8)
  line L126 (-495.3, 50.8) -> (-444.5, 50.8)
  line L127 (393.7, -50.8) -> (342.9, -50.8)
  line L128 (342.9, -50.8) -> (342.9, -101.6)
  line L129 (342.9, -101.6) -> (393.7, -101.6)
  line L130 (393.7, -101.6) -> (393.7, -50.8)
  line L131 (342.9, -50.8) -> (393.7, -101.6)
  circle A20 centre (368.3, -76.2) radius 15.875
  circle A21 centre (368.3, -381) radius 15.875
  line L132 (342.9, -406.4) -> (393.7, -406.4)
  line L133 (342.9, -355.6) -> (342.9, -406.4)
  line L134 (342.9, -355.6) -> (342.9, -406.4)
  line L135 (393.7, -406.4) -> (393.7, -355.6)
  line L136 (393.7, -355.6) -> (342.9, -355.6)
  line L137 (342.9, -355.6) -> (393.7, -355.6)
  line L138 (495.3, -50.8) -> (444.5, -50.8)
  line L139 (444.5, -50.8) -> (444.5, -101.6)
  line L140 (444.5, -101.6) -> (495.3, -101.6)
  line L141 (495.3, -101.6) -> (495.3, -50.8)
  line L142 (444.5, -101.6) -> (495.3, -50.8)
  line L143 (-393.7, -50.8) -> (-342.9, -50.8)
  line L144 (-342.9, -50.8) -> (-342.9, -101.6)
  line L145 (-342.9, -101.6) -> (-393.7, -101.6)
  line L146 (-393.7, -101.6) -> (-393.7, -50.8)
  line L147 (-495.3, -50.8) -> (-444.5, -50.8)
  line L148 (-444.5, -50.8) -> (-444.5, -101.6)
  line L149 (-444.5, -101.6) -> (-495.3, -101.6)
  line L150 (-495.3, -101.6) -> (-495.3, -50.8)
  line L151 (-342.9, -50.8) -> (-393.7, -101.6)
  line L152 (-444.5, -101.6) -> (-495.3, -50.8)
  circle A22 centre (-469.9, -76.2) radius 15.875
  circle A23 centre (-368.3, -76.2) radius 15.875
  circle A24 centre (469.9, -76.2) radius 15.875
  circle A25 centre (469.9, -381) radius 15.875
  line L153 (444.5, -406.4) -> (495.3, -406.4)
  line L154 (444.5, -355.6) -> (444.5, -406.4)
  line L155 (495.3, -406.4) -> (495.3, -355.6)
  line L156 (495.3, -355.6) -> (444.5, -355.6)
  line L157 (-444.5, -406.4) -> (-495.3, -406.4)
  line L158 (-495.3, -406.4) -> (-495.3, -355.6)
  line L159 (-444.5, -355.6) -> (-444.5, -406.4)
  line L160 (-495.3, -355.6) -> (-444.5, -355.6)
  circle A26 centre (-469.9, -381) radius 15.875
  circle A27 centre (-368.3, -381) radius 15.875
  line L161 (-342.9, -406.4) -> (-393.7, -406.4)
  line L162 (-393.7, -406.4) -> (-393.7, -355.6)
  line L163 (-342.9, -355.6) -> (-342.9, -406.4)
  line L164 (-342.9, -406.4) -> (-342.9, -355.6)
  line L165 (-393.7, -355.6) -> (-342.9, -355.6)
  line L166 (-342.9, -355.6) -> (-393.7, -355.6)
  line L167 (-342.9, -50.8) -> (-292.1, -50.8)
  line L168 (-292.1, -50.8) -> (-292.1, 0)
  line L169 (-292.1, 0) -> (-342.9, 0)
  line L170 (-342.9, 0) -> (-342.9, -50.8)
  line L171 (-342.9, 0) -> (-292.1, -50.8)
  circle A28 centre (-317.5, -25.4) radius 15.875
  circle A29 centre (-105.8333, -25.4) radius 15.875
  line L172 (-80.4333, -50.8) -> (-80.4333, 0)
  line L173 (-80.4333, 0) -> (-131.2333, 0)
  line L174 (-80.4333, -50.8) -> (-131.2333, -50.8)
  line L175 (-131.2333, -50.8) -> (-80.4333, -50.8)
  line L176 (-131.2333, 0) -> (-131.2333, -50.8)
  circle A30 centre (105.8333, -25.4) radius 15.875
  line L177 (131.2333, -50.8) -> (131.2333, 0)
  line L178 (131.2333, 0) -> (80.4333, 0)
  line L179 (131.2333, -50.8) -> (80.4333, -50.8)
  line L180 (80.4333, -50.8) -> (131.2333, -50.8)
  line L181 (80.4333, 0) -> (80.4333, -50.8)
  circle A31 centre (317.5, -25.4) radius 15.875
  line L182 (342.9, -50.8) -> (342.9, 0)
  line L183 (342.9, 0) -> (292.1, 0)
  line L184 (342.9, -50.8) -> (292.1, -50.8)
  line L185 (292.1, -50.8) -> (342.9, -50.8)
  line L186 (292.1, 0) -> (292.1, -50.8)
  line L187 (-495.3, -406.4) -> (-444.5, -457.2)
  line L188 (-393.7, -457.2) -> (-342.9, -406.4)
  line L189 (342.9, -406.4) -> (393.7, -457.2)
  line L190 (444.5, -457.2) -> (495.3, -406.4)
  line L191 (368.3, -431.8) -> (469.9, -431.8)
  line L192 (-469.9, -431.8) -> (-368.3, -431.8)
  line L193 (-425.45, -447.675) -> (-412.75, -447.675)
  line L194 (-412.75, -447.675) -> (-412.75, -415.925)
  line L195 (-412.75, -415.925) -> (-425.45, -415.925)
  line L196 (-425.45, -415.925) -> (-425.45, -447.675)
  line L197 (-425.45, -447.675) -> (-412.75, -415.925) construction
  line L198 (-412.75, -447.675) -> (-425.45, -415.925) construction
  line L199 (425.45, -447.675) -> (412.75, -447.675)
  line L200 (412.75, -447.675) -> (412.75, -415.925)
  line L201 (412.75, -415.925) -> (425.45, -415.925)
  line L202 (425.45, -415.925) -> (425.45, -447.675)
  line L203 (425.45, -447.675) -> (412.75, -415.925) construction
  line L204 (412.75, -447.675) -> (425.45, -415.925) construction
  point P0 (342.9, -152.4)
  point P1 (-342.9, -152.4)
  point P2 (342.9, -406.4)
  point P3 (-342.9, -406.4)
  point P4 (-131.2333, -50.8)
  point P5 (80.4333, -50.8)
  point P6 (292.1, -50.8)
  point P7 (-419.1, -431.8)
  point P8 (419.1, -431.8)
  dimension "d614" = 990.6
  dimension "d615" = 914.4
  dimension "d616" = 152.4
  dimension "d617" = 406.4
  dimension "d618" = 152.4
  dimension "d619" = 406.4
  dimension "d620" = 50.8
  dimension "d621" = 50.8
  dimension "d622" = 50.8
  dimension "d623" = 50.8
  dimension "d624" = 50.8
  dimension "d625" = 50.8
  dimension "d626" = 50.8
  dimension "d627" = 50.8
  dimension "d628" = 50.8
  dimension "d629" = 50.8
  dimension "d630" = 50.8
  dimension "d631" = 50.8
  dimension "d632" = 50.8
  dimension "d633" = 50.8
  dimension "d634" = 31.75
  dimension "d635" = 31.75
  dimension "d638" = 0
  dimension "d639" = 254
  dimension "d640" = 50.8
  dimension "d641" = 50.8
  dimension "d642" = 31.75
  dimension "d643" = 31.75
  dimension "d646" = 533.4
  dimension "d647" = 0
  dimension "d648" = 50.8
  dimension "d649" = 31.75
  dimension "d652" = 838.2
  dimension "d653" = 0
  dimension "d654" = 50.8
  dimension "d655" = 31.75
  dimension "d656" = 50.8
  dimension "d657" = 31.75
  dimension "d660" = 0
  dimension "d661" = -355.6
  dimension "d662" = 50.8
  dimension "d663" = 31.75
  dimension "d666" = 0
  dimension "d667" = -304.8
  dimension "d668" = 50.8
  dimension "d669" = 50.8
  dimension "d670" = 50.8
  dimension "d671" = 50.8
  dimension "d672" = 50.8
  dimension "d673" = 50.8
  dimension "d674" = 31.75
  dimension "d675" = 31.75
  dimension "d676" = 31.75
  dimension "d679" = 0
  dimension "d680" = -304.8
  dimension "d681" = 50.8
  dimension "d682" = 50.8
  dimension "d683" = 31.75
  dimension "d686" = 635
  dimension "d687" = 0
  dimension "d745" = 12.7
  dimension "d746" = 31.75
  dimension "d747" = 12.7
  dimension "d748" = 31.75
  constraint horizontal L0
  constraint perpendicular L0 L1
  constraint parallel L0 L2
  constraint parallel L1 L3
  constraint coincident L4 origin
  constraint coincident L5 origin
  constraint horizontal L6
  constraint vertical L7
  constraint horizontal L8
  constraint vertical L9
  constraint horizontal L10
  constraint vertical L11
  constraint horizontal L12
  constraint vertical L13
  constraint perpendicular L14 L15
  constraint parallel L14 L16
  constraint parallel L15 L17
  constraint perpendicular L18 L19
  constraint parallel L18 L20
  constraint parallel L19 L21
  constraint perpendicular L22 L23
  constraint parallel L22 L24
  constraint parallel L23 L25
  constraint perpendicular L26 L27
  constraint parallel L26 L28
  constraint parallel L27 L29
  constraint perpendicular L30 L31
  constraint parallel L30 L32
  constraint parallel L31 L33
  constraint perpendicular L34 L35
  constraint parallel L34 L36
  constraint parallel L35 L37
  constraint perpendicular L38 L39
  constraint parallel L38 L40
  constraint parallel L39 L41
  constraint perpendicular L42 L43
  constraint parallel L42 L44
  constraint parallel L43 L45
  constraint perpendicular L46 L47
  constraint parallel L46 L48
  constraint parallel L47 L49
  constraint perpendicular L50 L51
  constraint parallel L50 L52
  constraint parallel L51 L53
  constraint perpendicular L54 L55
  constraint parallel L54 L56
  constraint parallel L55 L57
  constraint perpendicular L58 L59
  constraint parallel L58 L60
  constraint parallel L59 L61
  constraint perpendicular L62 L63
  constraint parallel L62 L64
  constraint parallel L63 L65
  constraint coincident L56 L62.end
  constraint coincident L48 L62.end
  constraint perpendicular L66 L67
  constraint parallel L66 L68
  constraint parallel L67 L69
  constraint coincident L60 L66.end
  constraint coincident L48 L66.end
  constraint midpoint L70 A0.centre
  constraint midpoint L71 A1.centre
  constraint perpendicular L76 L77
  constraint parallel L76 L78
  constraint parallel L77 L79
  constraint perpendicular L80 L81
  constraint parallel L80 L82
  constraint parallel L81 L83
  constraint midpoint L85 A4.centre
  constraint midpoint L84 A5.centre
  constraint perpendicular L98 L99
  constraint parallel L98 L100
  constraint parallel L99 L101
  constraint coincident L20 L98.end
  constraint coincident L36 L98.end
  constraint midpoint L102 A12.centre
  constraint perpendicular L109 L110
  constraint parallel L109 L111
  constraint parallel L110 L112
  constraint midpoint L113 A16.centre
  constraint perpendicular L114 L115
  constraint parallel L114 L116
  constraint parallel L115 L117
  constraint midpoint L118 A17.centre
  constraint perpendicular L127 L128
  constraint parallel L127 L129
  constraint parallel L128 L130
  constraint midpoint L131 A20.centre
  constraint horizontal L138
  constraint vertical L139
  constraint horizontal L140
  constraint vertical L141
  constraint horizontal L143
  constraint vertical L144
  constraint horizontal L145
  constraint vertical L146
  constraint horizontal L147
  constraint vertical L148
  constraint horizontal L149
  constraint vertical L150
  constraint midpoint L152 A22.centre
  constraint midpoint L151 A23.centre
  constraint midpoint L142 A24.centre
  constraint horizontal L167
  constraint vertical L168
  constraint horizontal L169
  constraint vertical L170
  constraint midpoint L171 A28.centre
  constraint coincident P3 L27.end
  constraint midpoint L189 L191.start
  constraint midpoint L190 L191.end
  constraint midpoint L187 L192.start
  constraint midpoint L188 L192.end
  constraint horizontal L193
  constraint perpendicular L193 L194
  constraint parallel L193 L195
  constraint parallel L194 L196
  constraint coincident L197 P7
  constraint coincident L198 P7
  constraint midpoint L192 P7
  constraint horizontal L199
  constraint perpendicular L199 L200
  constraint parallel L199 L201
  constraint parallel L200 L202
  constraint coincident L203 P8
  constraint coincident L204 P8
  constraint midpoint L191 P8
  measures "d614" distance of L1.end L2.end
  measures "d615" distance of L0.end L1.end
  measures "d616" distance of L0.start L6.end
  measures "d617" distance of L0.start L8.end
  measures "d618" distance of L0.end L10.end
  measures "d619" distance of L0.end L12.end
  measures "d620" distance of L12.end L16.end
  measures "d621" distance of L1.end L20.end
  measures "d622" distance of L0.start L24.end
  measures "d623" distance of L0.end L28.end
  measures "d624" distance of L0.start L32.end
  measures "d625" distance of L1.end L36.end
  measures "d626" distance of L10.end L40.end
  measures "d627" distance of L6.end L44.end
  measures "d628" distance of L10.end P3
  measures "d629" distance of L11.end L52.end
  measures "d630" distance of L11.end L56.end
  measures "d631" distance of L7.end P6
  measures "d632" distance of P3 L64.end
  measures "d633" distance of P2 L68.end
  measures "d634" diameter of A0
  measures "d635" diameter of A1
  measures "d640" distance of L56.end L78.end
  measures "d641" distance of L62.end L82.end
  measures "d642" diameter of A4
  measures "d643" diameter of A5
  measures "d648" distance of L36.end L100.end
  measures "d649" diameter of A12
  measures "d654" distance of L107.start L111.end
  measures "d655" diameter of A16
  measures "d656" distance of L20.end L116.end
  measures "d657" diameter of A17
  measures "d662" distance of L43.end L129.end
  measures "d663" diameter of A20
  measures "d668" distance of L8.end L138.end
  measures "d669" distance of L8.end L140.end
  measures "d670" distance of L39.end L11.end
  measures "d671" distance of L39.end L145.end
  measures "d672" distance of L12.end L147.end
  measures "d673" distance of L12.end L149.end
  measures "d674" diameter of A22
  measures "d675" diameter of A23
  measures "d676" diameter of A24
  measures "d681" distance of L11.end L56.end
  measures "d682" distance of L11.end L169.end
  measures "d683" diameter of A28
  measures "d745" distance of L194.end L195.end
  measures "d746" distance of L193.end L194.end
  measures "d747" distance of L200.end L201.end
  measures "d748" distance of L199.end L200.end
extrude "Extrude15" add sketch "top-face" along normal blind 273.05 and the other way blind -266.7 separate body contours L0 L3 L6 L9 L22 L25 L30 L33 L190 | L0 L6 L22 L32 L44 L191 L199 L200 L202 | L32 L190 L191 | L3 L9 L24 L30 L32 L153 L154 L155 L156 | L24 L32 L153 L190 L191 | L44 L189 L191 | L0 L6 L7 L22 L23 L42 L45 L47 L58 L189 | L24 L32 L44 L191 L200 L201 L202 | L3 L9 L30 L32 L140 L156 | L24 L44 L132 L189 L191 | L3 L9 L30 L140 L141 L142 A24 | L7 L24 L42 L44 L58 L69 L132 L133 L134 L135 L136 L137 | L3 L8 L14 L15 L16 L30 L32 L119 L138 | L8 L14 L32 L138 L139 L142 A24 | L7 L42 L44 L58 L129 L136 L137 | L3 L16 L30 L32 L119 L123 L124 L125 | L8 L14 L16 L32 L43 L127 L182 | L142 A24 | L142 A24 | L8 L14 L43 L44 L127 L130 L131 A20 | L7 L42 L51 L58 L128 L129 L131 A20 | L3 L30 L32 L111 L125 | L131 A20 | L131 A20 | L3 L20 L30 L109 L110 L113 A16 | L32 L111 L112 L113 A16 | L14 L16 L50 L61 L182 L183 L184 L185 L186 | L2 L3 L18 L19 L20 L30 L31 L32 L107 L109 | L113 A16 | L113 A16 | L14 L16 L50 L177 L186 | L2 L18 L20 L32 L107 L108 | L14 L16 L50 L177 L178 L179 L180 L181 | L2 L18 L20 L105 L108 | L14 L16 L50 L172 L181 | L2 L18 L20 L105 L106 | L14 L16 L50 L172 L173 L174 L175 L176 | L0 L10 L11 L26 L27 L38 L41 L49 L54 L188 | L2 L18 L20 L103 L106 | L14 L16 L50 L79 L168 L176 | L0 L10 L26 L36 L40 L192 L193 L194 L196 | L40 L188 L192 | L11 L28 L38 L40 L54 L65 L161 L162 L163 L164 L165 L166 | L28 L40 L161 L188 L192 | L2 L18 L20 L103 L104 | L16 L168 L169 L171 A28 | L36 L187 L192 | L0 L1 L10 L13 L26 L29 L34 L35 L187 | L28 L36 L40 L192 L194 L195 L196 | L11 L38 L40 L54 L145 L165 L166 | L2 L18 L20 L100 L104 | L12 L14 L16 L36 L39 L143 L170 | L14 L50 L57 L167 L170 L171 A28 | L28 L36 L157 L187 L192 | L1 L13 L28 L34 L36 L157 L158 L159 L160 | L2 L18 L100 L101 L102 A12 | L20 L36 L98 L99 L102 A12 | L1 L12 L14 L16 L17 L34 L36 L120 L147 | L1 L16 L34 L36 L120 L121 L122 L126 | L12 L14 L39 L40 L143 L146 L151 A23 | L11 L38 L53 L54 L144 L145 L151 A23 | L171 A28 | L171 A28 | L1 L13 L34 L36 L149 L160 | L1 L20 L34 L114 L117 L118 A17 | L1 L2 L18 L20 L21 L34 L36 L37 L98 L114 | L36 L115 L116 L118 A17 | L102 A12 | L102 A12 | L12 L14 L36 L147 L148 L152 A22 | L1 L34 L36 L116 L126 | L151 A23 | L151 A23 | L1 L13 L34 L149 L150 L152 A22 | L118 A17 | L118 A17 | L152 A22 | L152 A22 | A13 | A14 | A15 | A18 | A19 | A21 | A25 | A26 | A27 | A29 | A30 | A31 makes body 5